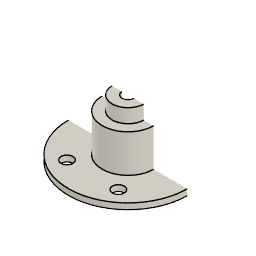
Brodie Stem Nut (Autodesk Fusion 360 design; units mm, degrees)
Autodesk Fusion 360 part; units mm, degrees
sketch "Sketch1" plane through (0, 0, 0) normal (0, 0, 1) x (1, 0, 0)
  circle A0 centre (0, 0) radius 15
  dimension "d1" = 30
  constraint coincident A0.centre origin
  measures "d1" diameter of A0
extrude "Extrude1" add sketch "Sketch1" along normal blind 1.5
sketch "Sketch2" plane through (0, 0, 1.5) normal (0, 0, 1) x (-1, 0, 0)
  circle A0 centre (0, 0) radius 15
  circle A1 centre (0, -11) radius 1.5
  circle A2 centre (10.4616, -3.3992) radius 1.5
  circle A3 centre (6.4656, 8.8992) radius 1.5
  circle A4 centre (-6.4656, 8.8992) radius 1.5
  circle A5 centre (-10.4616, -3.3992) radius 1.5
  dimension "d4" = 3
  dimension "d6" = 360
  measures "d4" diameter of A1
extrude "Extrude2" cut sketch "Sketch2" against normal blind 10 contours A1 | A2 | A3 | A4 | A5
sketch "Sketch3" plane through (0, 0, 1.5) normal (0, 0, 1) x (-1, 0, 0)
  circle A0 centre (-6.4656, 8.8992) radius 1.5
  circle A1 centre (-10.4616, -3.3992) radius 1.5
  circle A2 centre (6.4656, 8.8992) radius 1.5
  circle A3 centre (0, -11) radius 1.5
  circle A4 centre (10.4616, -3.3992) radius 1.5
  circle A5 centre (0, 0) radius 15
  circle A6 centre (0, 0) radius 6.5
  dimension "d9" = 13
  constraint concentric A5 A6
  measures "d9" diameter of A6
extrude "Extrude3" add sketch "Sketch3" along normal blind 9.5 contours A6
sketch "Sketch4" plane through (0, 0, 11) normal (0, 0, 1) x (-1, 0, 0)
  circle A0 centre (0, 0) radius 6.5
  circle A1 centre (0, 0) radius 4
  dimension "d12" = 8
  constraint coincident A0.centre A1.centre
  measures "d12" diameter of A1
extrude "Extrude4" add sketch "Sketch4" along normal blind 3.5 contours A1
extrude "Extrude5" add 1 faces at (-1.8435, -0.6041, 0) along direction (0, 0, -1) blind 0.5
sketch "Sketch5" plane through (0, 0, -0.5) normal (0, 0, -1) x (1, 0, 0)
  circle A0 centre (6.4656, 8.8992) radius 1.5
  circle A1 centre (10.4616, -3.3992) radius 1.5
  circle A2 centre (-6.4656, 8.8992) radius 1.5
  circle A3 centre (0, -11) radius 1.5
  circle A4 centre (-10.4616, -3.3992) radius 1.5
  circle A5 centre (0, 0) radius 15
  circle A6 centre (0, 0) radius 3
  constraint concentric A5 A6
extrude "Extrude6" cut sketch "Sketch5" against normal blind 2 contours A6
move_body "Move1" bodies 1 to x (1, 0, 0) y (0, 1, 0) z (0, 0, 1) at (0, 0, 0.5)
sketch "Sketch6" plane through (0, 0, 15) normal (0, 0, 1) x (-1, 0, 0)
  circle A0 centre (0, 0) radius 4
  circle A1 centre (0, 0) radius 1.5
  dimension "d19" = 3
  constraint concentric A0 A1
  measures "d19" diameter of A1
extrude "Extrude7" cut sketch "Sketch6" against normal blind 100 contours A1
ref_plane "WorkPlane1" through (0, 0, 9.5) normal (0, 0, 1) x (1, 0, 0)
sketch "Sketch7" plane through (0, 0, 9.5) normal (0, 0, 1) x (1, 0, 0)
  line L0 (2.8, 1.6166) -> (0, 3.2332)
  line L1 (0, 3.2332) -> (-2.8, 1.6166)
  line L2 (-2.8, 1.6166) -> (-2.8, -1.6166)
  line L3 (-2.8, -1.6166) -> (0, -3.2332)
  line L4 (0, -3.2332) -> (2.8, -1.6166)
  line L5 (2.8, -1.6166) -> (2.8, 1.6166)
  dimension "d28" = 2.8
  measures "d28" distance of origin L5
extrude "Extrude10" cut sketch "Sketch7" against normal blind 4
sketch "Sketch8" plane through (0, 0, 0) normal (0, 0, -1) x (1, 0, 0)
  circle A0 centre (0, 0) radius 3
  circle A1 centre (6.4656, 8.8992) radius 1.5
  circle A2 centre (10.4616, -3.3992) radius 1.5
  circle A3 centre (-6.4656, 8.8992) radius 1.5
  circle A4 centre (0, -11) radius 1.5
  circle A5 centre (-10.4616, -3.3992) radius 1.5
  circle A6 centre (0, 0) radius 15
extrude "Extrude11" cut sketch "Sketch8" against normal blind 0.5
move_body "Move2" bodies 1 to x (1, 0, 0) y (0, 1, 0) z (0, 0, 1) at (0, 0, -0.5)
extrude "Extrude12" cut 1 faces at (2.4832, 0.2236, 1.5) along direction (0, 0, 1) blind 0.5
